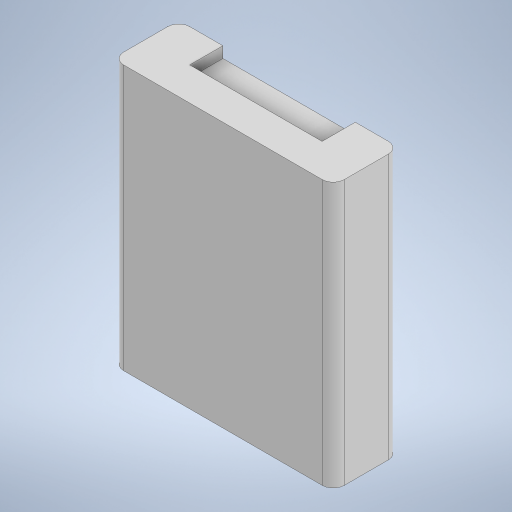
# Autodesk Inventor part: 2 Stütze
Saved by Autodesk Inventor 2023 (Build 270158000, 158)
## iProperties
Created: 2024-02-04
Part Number: 2 Stütze
Material: Generisch
Document SubType Name: Modeling
Designer: jefar
Density: 1 g/cm^3
Appearance: Vorgabe
Author: jefar
Autodesk Inventor part; units mm, degrees
ref_plane "YZ Plane" through (0, 0, 0) normal (1, 0, 0) x (0, 1, 0)
ref_plane "XZ Plane" through (0, 0, 0) normal (0, 1, 0) x (-1, 0, 0)
ref_plane "XY Plane" through (0, 0, 0) normal (0, 0, 1) x (1, 0, 0)
sketch "Skizze1" plane through (0, 0, 0) normal (0, 0, 1) x (1, 0, 0)
  line L0 (-7000, 0) -> (7000, 0) construction
  line L1 (0, -8400) -> (0, 8400) construction
  line L2 (-5000, -6000) -> (5000, -6000)
  line L3 (5000, -6000) -> (5000, 6000)
  line L4 (5000, 6000) -> (-5000, 6000)
  line L5 (-5000, 6000) -> (-5000, -6000)
  line L6 (-5000, -6000) -> (5000, 6000) construction
  line L7 (5000, -6000) -> (-5000, 6000) construction
  point P0 (0, 0)
  dimension "d0" = 10000
  dimension "d1" = 12000
  constraints: 12 end point, 2 midpoint, 2 parallel, 1 horizontal, 1 perpendicular
  measures "d0" distance of L4.end L3.end
  measures "d1" distance of L3.end L2.end
extrude "Extrusion1" add sketch "Skizze1" along normal blind 3000
sketch "Skizze2" plane through (-5000, 6000, 0) normal (0, 1, 0) x (1, 0, 0)
  line L0 (5000, 0) -> (2000, 0)
  line L1 (2000, 0) -> (2000, -1505)
  line L2 (2000, -1505) -> (5000, -1505)
  line L3 (5000, 0) -> (8000, 0)
  line L4 (8000, 0) -> (8000, -1505)
  line L5 (8000, -1505) -> (5000, -1505)
  dimension "d4" = 3000
  dimension "d5" = 1505
  dimension "d6" = 3000
  constraints: 12 end point, 2 horizontal, 2 parallel, 2 perpendicular
  measures "d4" distance of L2.end L1.end
  measures "d5" distance of L0.end L1.end
  measures "d6" distance of L4.end L5.end
extrude "Extrusion2" cut sketch "Skizze2" against normal blind 500
fillet "Rundung1" radius 500 4 edges at (5000, 0, 0) (5000, 0, 3000) (-5000, 0, 0) (-5000, 0, 3000)
